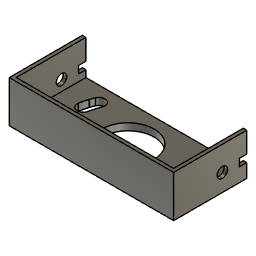
Wall Mount v20 (Autodesk Fusion 360 design; units mm, degrees)
Autodesk Fusion 360 part; units mm, degrees
note: some values were not read from the file. Chosen so that the rebuilt part matches the saved one: which face or edge a step refers to. Set by a fixed rule: which sketch regions a step uses.
sketch "Schizzo1" plane through (0, 0, 0) normal (0, 1, 0) x (1, 0, 0)
  line L0 (-116.8818, -54.9248) -> (-26.8818, -54.9248) construction
  line L1 (-26.8818, -54.9248) -> (-26.8818, -30.9248) construction
  line L2 (-26.8818, -30.9248) -> (-116.8818, -30.9248) construction
  line L3 (-116.8818, -30.9248) -> (-116.8818, -54.9248) construction
  line L4 (-119.0818, -54.9248) -> (-24.6818, -54.9248)
  line L5 (-24.6818, -54.9248) -> (-24.6818, -30.9248)
  line L6 (-24.6818, -30.9248) -> (-119.0818, -30.9248)
  line L7 (-119.0818, -30.9248) -> (-119.0818, -54.9248)
  line L8 (-71.8818, -54.9248) -> (-71.8818, -30.9248) construction
  line L9 (-71.8818, -54.9248) -> (-71.8818, -30.9248) construction
  line L10 (-26.6818, -54.9248) -> (-26.6818, -30.9248)
  line L11 (-117.0818, -54.9248) -> (-117.0818, -24.9248)
  line L12 (-119.0818, -34.9248) -> (-24.6818, -34.9248)
  line L13 (-119.0818, -54.9248) -> (-24.6818, -54.9248)
  line L14 (-24.6818, -54.9248) -> (-24.6818, -56.9248)
  line L15 (-24.6818, -56.9248) -> (-119.0818, -56.9248)
  line L16 (-119.0818, -56.9248) -> (-119.0818, -54.9248)
  dimension "d1" = 90
  dimension "d2" = 24
  dimension "d3" = 94.4
  dimension "d5" = 2
  dimension "d6" = 2
  dimension "d7" = 4
  dimension "d37" = 2
  constraint horizontal L0
  constraint vertical L1
  constraint horizontal L2
  constraint vertical L3
  constraint horizontal L4
  constraint vertical L5
  constraint horizontal L6
  constraint vertical L7
  constraint midpoint L0 L8.start
  constraint midpoint L2 L8.end
  constraint midpoint L4 L8.start
  constraint midpoint L6 L8.end
  constraint collinear L8 L9
  constraint collinear L2 L6
  constraint collinear L0 L4
  constraint coincident L4 L10.start
  constraint perpendicular L2 L10
  constraint coincident L6 L10.end
  constraint coincident L0 L11.start
  constraint perpendicular L2 L11
  constraint coincident L7 L12.start
  constraint coincident L5 L12.end
  constraint perpendicular L5 L12
  constraint horizontal L13
  constraint vertical L14
  constraint horizontal L15
  constraint vertical L16
  constraint collinear L5 L14
  measures "d1" distance of L0.start L0.end
  measures "d2" distance of L0.start L2.end
  measures "d3" distance of L4.start L4.end
  measures "d5" distance of L7 L11
  measures "d6" distance of L5 L10
  measures "d7" distance of L2 L12
  measures "d37" distance of L4 L15
extrude "Estrusione1" add sketch "Schizzo1" along normal blind 2 contours L4 L7 L11 L12 L13 | L4 L10 L11 L12 L13 | L6 L7 L11 L12 | L4 L5 L10 L12 L13 | L6 L10 L11 L12 | L5 L6 L10 L12
extrude "Estrusione2" add sketch "Schizzo1" along normal blind 42 contours L4 L7 L11 L12 L13 | L6 L7 L11 L12 | L4 L5 L10 L12 L13 | L6 L10 L11 L12 | L5 L6 L10 L12
sketch "Schizzo3" plane through (0, 0, 30.9248) normal (0, 0, -1) x (1, 0, 0)
  line L0 (-24.6818, 0) -> (-119.0818, 0)
  line L1 (-119.0818, 0) -> (-119.0818, -42)
  line L2 (-119.0818, -42) -> (-24.6818, -42)
  line L3 (-24.6818, -42) -> (-24.6818, 0)
  line L4 (-24.6818, -42) -> (-119.0818, -42) construction
  line L5 (-119.0818, -42) -> (-119.0818, 0) construction
  line L6 (-119.0818, 0) -> (-24.6818, 0) construction
  line L7 (-24.6818, 0) -> (-24.6818, -42) construction
  line L8 (-24.6818, -21) -> (-119.0818, -21) construction
  line L9 (-71.8818, -42) -> (-71.8818, 0) construction
  circle A0 centre (-71.8818, -21) radius 15
  line L10 (-24.6818, -31) -> (-119.0818, -31) construction
  line L11 (-41.8818, -31) -> (-41.8818, -11) construction
  circle A1 centre (-41.8818, -31) radius 3.5
  circle A2 centre (-41.8818, -11) radius 3.5
  circle A3 centre (-101.8818, -31) radius 3.5
  circle A4 centre (-101.8818, -11) radius 3.5
  line L12 (-119.0818, -11) -> (-24.6818, -11) construction
  line L13 (-71.8818, -21) -> (-42.7729, -33.356) construction
  line L14 (-71.8818, -21) -> (-36.6301, -21) construction
  line L15 (-71.8818, -21) -> (-41.8818, -31) construction
  circle A5 centre (-42.7729, -33.356) radius 3.5
  line L16 (-71.8818, -21) -> (-40.7394, -26.4912) construction
  circle A6 centre (-40.7394, -26.4912) radius 3.5
  circle A7 centre (-42.7729, -8.644) radius 3.5
  circle A8 centre (-40.7394, -15.5088) radius 3.5
  circle A9 centre (-100.9907, -33.356) radius 3.5
  circle A10 centre (-103.0242, -26.4912) radius 3.5
  circle A11 centre (-103.0242, -15.5088) radius 3.5
  circle A12 centre (-100.9907, -8.644) radius 3.5
  arc A13 (-39.5361, -34.6877) -> (-37.2861, -27.0607) centre (-71.8818, -21) ccw
  arc A14 (-45.9946, -31.9884) -> (-44.1863, -25.8835) centre (-71.8818, -21) ccw
  arc A15 (-37.2861, -14.9393) -> (-39.5361, -7.3123) centre (-71.8818, -21) ccw
  arc A16 (-44.1863, -16.1165) -> (-45.9946, -10.0116) centre (-71.8818, -21) ccw
  arc A17 (-99.5773, -25.8835) -> (-97.7689, -31.9884) centre (-71.8818, -21) ccw
  arc A18 (-106.4775, -27.0607) -> (-104.2275, -34.6877) centre (-71.8818, -21) ccw
  arc A19 (-97.7689, -10.0116) -> (-99.5773, -16.1165) centre (-71.8818, -21) ccw
  arc A20 (-104.2275, -7.3123) -> (-106.4775, -14.9393) centre (-71.8818, -21) ccw
  dimension "d21" = 30
  dimension "d22" = 10
  dimension "d23" = 7
  dimension "d24" = 7
  dimension "d25" = 30
  dimension "d40" = 10
  dimension "d44" = 23
  dimension "d45" = 7
  dimension "d46" = 10
  dimension "d47" = 7
  constraint horizontal L4
  constraint vertical L5
  constraint horizontal L6
  constraint vertical L7
  constraint coincident L0.end L1.start
  constraint coincident L2.end L3.start
  constraint midpoint L7 L8.start
  constraint midpoint L5 L8.end
  constraint midpoint L4 L9.start
  constraint midpoint L6 L9.end
  constraint midpoint L8 A0.centre
  constraint coincident L7 L10.start
  constraint coincident L5 L10.end
  constraint perpendicular L5 L10
  constraint perpendicular L8 L11
  constraint symmetric L9 A1 A3
  constraint symmetric L9 A2 A4
  constraint coincident L5 L12.start
  constraint coincident L7 L12.end
  constraint perpendicular L7 L12
  constraint coincident L11.end L12
  constraint coincident L10 L11.start
  constraint coincident L11.end A2.centre
  constraint horizontal L14
  constraint coincident A0.centre L13.start
  constraint coincident L11.start A1.centre
  constraint equal L13 L15
  constraint coincident L13.end A5.centre
  constraint coincident L16.end A6.centre
  constraint equal L15 L16
  constraint symmetric L14 A5 A7
  constraint symmetric L14 A6 A8
  constraint symmetric L9 A5 A9
  constraint symmetric L9 A6 A10
  constraint symmetric L9 A7 A12
  constraint symmetric L9 A8 A11
  constraint coincident A6 A13.end
  constraint coincident A5 A13.start
  constraint coincident A5 A14.start
  constraint coincident L13 A14.start
  constraint coincident L16 A14.end
  constraint symmetric L8 A13.start A15.end
  constraint symmetric L8 A13.end A15.start
  constraint symmetric L8 A13 A15
  constraint symmetric L8 A14.start A16.end
  constraint symmetric L8 A14.end A16.start
  constraint symmetric L8 A14 A16
  constraint symmetric L9 A13.start A18.end
  constraint symmetric L9 A13.end A18.start
  constraint symmetric L9 A13 A18
  constraint symmetric L9 A14.start A17.end
  constraint symmetric L9 A14.end A17.start
  constraint symmetric L9 A14 A17
  constraint symmetric L9 A15.end A20.start
  constraint symmetric L9 A15.start A20.end
  constraint symmetric L9 A15 A20
  constraint symmetric L9 A16.end A19.start
  constraint symmetric L9 A16.start A19.end
  constraint symmetric L9 A16 A19
  measures "d21" diameter of A0
  measures "d22" distance of L8 L10
  measures "d23" diameter of A1
  measures "d24" diameter of A2
  measures "d25" distance of L9 L11
  measures "d40" distance of L8 L12
  measures "d44" angle of L13 L14
  measures "d45" diameter of A5
  measures "d46" angle of L14 L16
  measures "d47" diameter of A6
extrude "Estrusione4" cut sketch "Schizzo3" against normal blind 5 contours A0 | A1 A5 A6 | A1 A6 | A1 A6 A13 | A1 A6 | A1 A5 A13 | A1 A6 A14 | A1 A5 | A1 A5 | A1 A5 A14 | A2 A7 A8 | A2 A8 A15 | A2 A7 A15 | A2 A8 | A2 A8 | A2 A7 | A2 A7 | A2 A8 A16 | A2 A7 A16 | A3 A9 A10 | A3 A9 A17 | A3 A10 A17 | A3 A10 | A3 A9 | A3 A9 | A3 A10 | A3 A9 A18 | A3 A10 A18 | A4 A11 A12 | A4 A12 A19 | A4 A12 | A4 A12 | A4 A11 A19 | A4 A11 A20 | A4 A12 A20 | A4 A11 | A4 A11
sketch "Schizzo4" plane through (-24.6818, 0, 0) normal (1, 0, 0) x (0, 1, 0)
  line L0 (0, 54.9248) -> (0, 30.9248)
  line L1 (0, 30.9248) -> (42, 30.9248)
  line L2 (42, 30.9248) -> (42, 54.9248)
  line L3 (42, 54.9248) -> (0, 54.9248)
  circle A0 centre (28, 40.9248) radius 3
  line L4 (0, 54.9248) -> (42, 54.9248) construction
  line L5 (42, 54.9248) -> (42, 30.9248) construction
  line L6 (42, 30.9248) -> (0, 30.9248) construction
  line L7 (0, 30.9248) -> (0, 54.9248) construction
  line L8 (0, 40.9248) -> (42, 40.9248) construction
  line L9 (42, 38.8248) -> (37.8, 38.8248)
  line L10 (37.8, 38.8248) -> (37.8, 43.0248)
  line L11 (37.8, 43.0248) -> (42, 43.0248)
  line L12 (42, 43.0248) -> (42, 38.8248)
  line L13 (42, 38.8248) -> (37.8, 43.0248) construction
  line L14 (37.8, 38.8248) -> (42, 43.0248) construction
  point P0 (39.9, 40.9248)
  dimension "d28" = 6
  dimension "d35" = 10
  dimension "d36" = 28
  dimension "d38" = 4.2
  dimension "d39" = 4.2
  constraint horizontal L4
  constraint vertical L5
  constraint horizontal L6
  constraint vertical L7
  constraint coincident L0.start L3.end
  constraint coincident L1.end L2.start
  constraint coincident L7 L8.start
  constraint coincident L5 L8.end
  constraint perpendicular L5 L8
  constraint coincident A0.centre L8
  constraint horizontal L9
  constraint perpendicular L9 L10
  constraint parallel L9 L11
  constraint parallel L10 L12
  constraint coincident L13 P0
  constraint coincident L14 P0
  constraint coincident L8 P0
  constraint collinear L5 L12
  measures "d28" diameter of A0
  measures "d35" distance of L6 L8
  measures "d36" distance of A0.centre L7
  measures "d38" distance of L10.end L11.end
  measures "d39" distance of L9.end L10.end
extrude "Estrusione5" cut sketch "Schizzo4" against normal blind 5 contours L2 L9 L10 L11 L12 | A0
extrude "Estrusione6" cut sketch "Schizzo4" against normal blind 5 from surface at -92.4 contours L2 L9 L10 L11 L12 | A0
sketch "Schizzo5" plane through (0, 42, 0) normal (0, 1, 0) x (-1, 0, 0)
  line L0 (119.0818, 38.8248) -> (117.0818, 38.8248)
  line L1 (117.0818, 38.8248) -> (117.0818, 34.9248)
  line L2 (117.0818, 34.9248) -> (26.6818, 34.9248)
  line L3 (26.6818, 34.9248) -> (26.6818, 38.8248)
  line L4 (26.6818, 38.8248) -> (24.6818, 38.8248)
  line L5 (24.6818, 38.8248) -> (24.6818, 30.9248)
  line L6 (24.6818, 30.9248) -> (119.0818, 30.9248)
  line L7 (119.0818, 30.9248) -> (119.0818, 38.8248)
  line L8 (24.6818, 38.8248) -> (119.0818, 38.8248) construction
  line L9 (119.0818, 38.8248) -> (119.0818, 30.9248) construction
  line L10 (119.0818, 30.9248) -> (24.6818, 30.9248) construction
  line L11 (24.6818, 30.9248) -> (24.6818, 38.8248) construction
  line L12 (24.6818, 32.9248) -> (119.0818, 32.9248)
  line L13 (119.0818, 32.9248) -> (119.0818, 30.9248)
  line L14 (119.0818, 30.9248) -> (24.6818, 30.9248)
  line L15 (24.6818, 30.9248) -> (24.6818, 32.9248)
  dimension "d41" = 2
  constraint horizontal L8
  constraint vertical L9
  constraint horizontal L10
  constraint vertical L11
  constraint coincident L6.end L7.start
  constraint coincident L4.end L5.start
  constraint horizontal L12
  constraint vertical L13
  constraint horizontal L14
  constraint vertical L15
  constraint collinear L11 L15
  measures "d41" distance of L12 L14
extrude "Estrusione7" [rolled back] along distance -5 taper angle 0
equation "d3 = 4 mm + 90 mm + 0.4 mm"
equation "d6 = d5"
equation "d24 = d23"
equation "d38 = 4 mm + 0.2 mm"
equation "d39 = 4 mm + 0.2 mm"
equation "d40 = d22"
equation "d45 = d23"
equation "d47 = d23"
